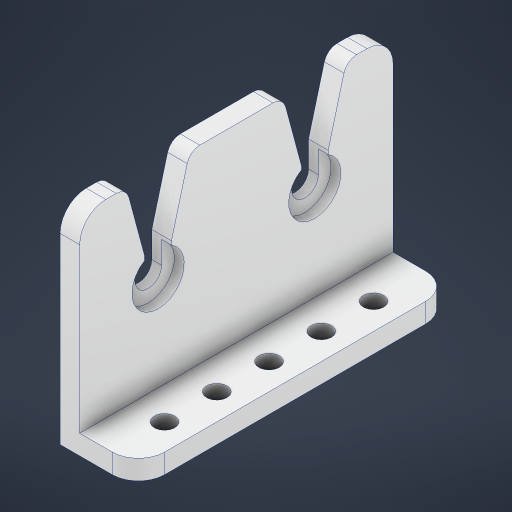
# Autodesk Inventor part: BUMP_006_Bigbracket
Saved by Autodesk Inventor 2024.2 (Build 282272000, 272)
## iProperties
Created: 2024-08-10
Part Number: BUMP_006_Bigbracket
Material: Aluminum 6061
Document SubType Name: Modeling
Designer: Bryan
Density: 2.7 g/cm^3
Appearance: Aluminum - Flat
Author: Bryan
Autodesk Inventor part; units mm, degrees
ref_plane "YZ Plane" through (0, 0, 0) normal (1, 0, 0) x (0, 1, 0)
ref_plane "XZ Plane" through (0, 0, 0) normal (0, 1, 0) x (-1, 0, 0)
ref_plane "XY Plane" through (0, 0, 0) normal (0, 0, 1) x (1, 0, 0)
sketch "Sketch1" plane through (0, 0, 0) normal (0, 0, 1) x (1, 0, 0)
  line L0 (0, 0) -> (0, 50.8)
  line L1 (0, 50.8) -> (4.7625, 50.8)
  line L2 (4.7625, 50.8) -> (4.7625, 4.7625)
  line L3 (4.7625, 4.7625) -> (19.05, 4.7625)
  line L4 (19.05, 4.7625) -> (19.05, 0)
  line L5 (19.05, 0) -> (0, 0)
  dimension "d0" = 4.7625
  dimension "d1" = 19.05
  dimension "d2" = 50.8
  dimension "d3" = 4.7625
  constraints: 12 end point, 3 horizontal, 3 vertical
  measures "d0" distance of L0.end L1.end
  measures "d1" distance of L4.end L0.start
  measures "d2" distance of L0.start L0.end
  measures "d3" distance of L3.end L4.end
extrude "Extrusion1" add sketch "Sketch1" along normal blind 76.2
sketch "Sketch2" plane through (4.7625, 4.7625, 0) normal (1, 0, 0) x (0, 0, -1)
  circle A0 centre (-57.15, 23.0187) radius 3.2512
  circle A1 centre (-19.05, 23.0187) radius 3.2512
  line L0 (-76.2, 0) -> (-76.2, 46.0375) projected
  line L1 (0, 0) -> (0, 46.0375) projected
  line L2 (-60.4012, 23.0187) -> (-60.4012, 29.3687)
  line L3 (-60.4012, 29.3687) -> (-64.8676, 46.0375)
  line L4 (0, 46.0375) -> (-76.2, 46.0375) projected
  line L5 (-53.8988, 23.0187) -> (-53.8988, 29.3687)
  line L6 (-53.8988, 29.3687) -> (-49.4324, 46.0375)
  line L7 (-22.3012, 23.0187) -> (-22.3012, 29.3687)
  line L8 (-22.3012, 29.3687) -> (-26.7676, 46.0375)
  line L9 (-11.3324, 46.0375) -> (-15.7988, 29.3687)
  line L10 (-15.7988, 29.3687) -> (-15.7988, 23.0187)
  point P0 (0, -4.7625)
  point P1 (-76.2, 23.0187)
  point P2 (0, 23.0187)
  point P3 (-76.2, 23.0187)
  dimension "d6" = 6.5024
  dimension "d7" = 6.5024
  dimension "d8" = 19.05
  dimension "d9" = 38.1
  dimension "d10" = 19.05
  dimension "d11" = 6.35
  dimension "d12" = 165
  constraints: 16 end point, 6 equal length, 4 point on circle, 4 point on line, 4 tangent, 3 midpoint, 3 vertical, 2 centre point, 2 horizontal alignment, 1 parallel
  measures "d6" diameter of A0
  measures "d7" diameter of A1
  measures "d8" distance from line of L0 A0.centre
  measures "d9" distance of A1.centre A0.centre
  measures "d10" distance of point (0, 23.019) A1.centre
  measures "d11" distance of L2.start L2.end
  measures "d12" angle of L3 L2
extrude "Extrusion2" cut sketch "Sketch2" against normal blind 76.2
sketch "Sketch3" plane through (4.7625, 4.7625, 0) normal (1, 0, 0) x (0, 0, -1)
  arc A0 (-22.3012, 23.0187) -> (-15.7988, 23.0187) centre (-19.05, 23.0187) ccw projected
  circle A1 centre (-19.05, 23.0187) radius 6.35
  arc A2 (-60.4012, 23.0187) -> (-53.8988, 23.0187) centre (-57.15, 23.0187) ccw projected
  circle A3 centre (-57.15, 23.0187) radius 6.35
  point P0 (0, -4.7625)
  dimension "d15" = 12.7
  dimension "d16" = 12.7
  constraints: 2 centre point, 2 coincident
  measures "d15" diameter of A1
  measures "d16" diameter of A3
extrude "Extrusion3" cut sketch "Sketch3" against normal blind 2.3813
fillet "Fillet1" radius 3.175 4 edges at (2.3813, 50.8, 64.8676) (2.3813, 50.8, 49.4324) (2.3813, 50.8, 26.7676) (2.3813, 50.8, 11.3324)
sketch "Sketch4" plane through (4.7625, 4.7625, 0) normal (0, 1, 0) x (1, 0, 0)
  circle A0 centre (7.9375, -63.5) radius 2.4892
  line L0 (14.2875, -76.2) -> (0, -76.2) projected
  line L1 (14.2875, 0) -> (14.2875, -76.2) projected
  circle A1 centre (7.9375, -50.8) radius 2.4892
  circle A2 centre (7.9375, -38.1) radius 2.4892
  circle A3 centre (7.9375, -25.4) radius 2.4892
  circle A4 centre (7.9375, -12.7) radius 2.4892
  circle A5 centre (7.9375, 0) radius 2.4892 construction
  line L2 (-4.7625, -67.3038) -> (-4.7625, -76.2) projected
  line L3 (-4.7625, -67.3038) -> (-4.7625, -64.237) projected
  line L4 (-4.7625, -60.4012) -> (-4.7625, -53.8988) projected
  line L5 (0, -64.237) -> (-4.7625, -64.237) projected
  line L6 (0, -60.4012) -> (0, -64.237) projected
  line L7 (0, -60.4012) -> (-4.7625, -60.4012) projected
  line L8 (-4.7625, -64.237) -> (-4.7625, -60.4012) projected
  point P0 (-4.7625, 0)
  point P1 (7.1437, -76.2)
  dimension "d20" = 4.9784
  dimension "d21" = 12.7
  dimension "d24" = 12.7
  dimension "d33" = 12.7
  constraints: 6 centre point, 1 midpoint, 1 vertical, 10 other
  measures "d20" diameter of A0
  measures "d21" distance from line of L0 A0.centre
  measures "d24" distance of A0.centre A1.centre
  measures "d33" distance from line of L2 A0.centre
extrude "Extrusion4" cut sketch "Sketch4" against normal through all contours A0 | A1 | A2 | A3 | A4
fillet "Fillet2" radius 6.35 4 edges at (19.05, 2.3813, 76.2) (19.05, 2.3813, 0) (2.3813, 50.8, 76.2) (2.3813, 50.8, 0)
equation "\"d8\" = d10"
body "Solid1"
